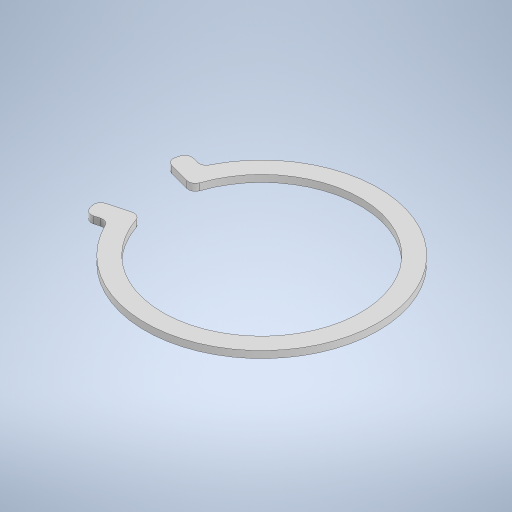
# Autodesk Inventor part: BearingRing
Saved by Autodesk Inventor 2023 (Build 270158030, 158C)
## iProperties
Created: 2024-10-25
Part Number: BearingRing
Material: Generic
Document SubType Name: Modeling
Designer: lvrectanus0
Density: 1 g/cm^3
Appearance: Default
Author: lvrectanus0
Autodesk Inventor part; units mm, degrees
ref_plane "YZ Plane" through (0, 0, 0) normal (1, 0, 0) x (0, 1, 0)
ref_plane "XZ Plane" through (0, 0, 0) normal (0, 1, 0) x (-1, 0, 0)
ref_plane "XY Plane" through (0, 0, 0) normal (0, 0, 1) x (1, 0, 0)
sketch "Sketch1" plane through (0, 0, 0) normal (0, 1, 0) x (-1, 0, 0)
  arc A0 (13.5292, 4.5927) -> (13.5292, -4.5927) centre (0, 0) ccw
  arc A1 (15.0656, 7.4961) -> (15.0656, -7.4961) centre (0, 0) ccw
  line L0 (14.735, -3.9482) -> (16.2541, -4.3553)
  line L1 (0, 0) -> (16.8275, 0) construction
  line L2 (14.735, 3.9482) -> (16.2541, 4.3553)
  line L3 (0, 0) -> (16.8275, 0) construction
  line L4 (16.2541, 4.3553) -> (17.7416, 4.7539)
  line L5 (18.4487, 5.9786) -> (18.309, 6.5002)
  line L6 (17.0842, 7.2073) -> (16.2197, 6.9757)
  line L7 (16.2541, -4.3553) -> (17.7416, -4.7539)
  line L8 (18.4487, -5.9786) -> (18.309, -6.5002)
  line L9 (17.0842, -7.2073) -> (16.2197, -6.9757)
  arc A2 (13.5292, 4.5927) -> (14.735, 3.9482) centre (14.4761, 4.9141) ccw
  arc A3 (17.7416, 4.7539) -> (18.4487, 5.9786) centre (17.4828, 5.7198) ccw
  arc A4 (18.309, 6.5002) -> (17.0842, 7.2073) centre (17.3431, 6.2414) ccw
  arc A5 (15.0656, 7.4961) -> (16.2197, 6.9757) centre (15.9609, 7.9416) ccw
  arc A6 (14.735, -3.9482) -> (13.5292, -4.5927) centre (14.4761, -4.9141) ccw
  arc A7 (18.4487, -5.9786) -> (17.7416, -4.7539) centre (17.4828, -5.7198) ccw
  arc A8 (17.0842, -7.2073) -> (18.309, -6.5002) centre (17.3431, -6.2414) ccw
  arc A9 (16.2197, -6.9757) -> (15.0656, -7.4961) centre (15.9609, -7.9416) ccw
  point P0 (13.8007, 3.6979)
  point P1 (13.8007, -3.6979)
  point P2 (18.7076, 5.0127)
  point P3 (18.0502, 7.4661)
  point P4 (15.4105, 6.7588)
  point P5 (18.7076, -5.0127)
  point P6 (18.0502, -7.4661)
  point P7 (15.4105, -6.7588)
  dimension "d0" = 28.575
  dimension "d1" = 2.54
  dimension "d2" = 15
  dimension "d3" = 15
  dimension "d4" = 2.54
  dimension "d5" = 2.54
  dimension "d6" = 90
  dimension "d7" = 2.54
  dimension "d8" = 2.54
  dimension "d9" = 1
  dimension "d10" = 1
  constraints: 27 point on circle, 20 end point, 16 tangent, 12 point on line, 10 centre point, 6 equal radius, 3 perpendicular, 2 horizontal, 1 coincident
  measures "d0" diameter of A0
  measures "d1" radial gap between concentric circles of A0 A1
  measures "d2" angle of L0 L1
  measures "d3" angle of L3 L2
  measures "d4" distance of L2.end point (18.708, 5.013)
  measures "d5" distance of point (18.708, 5.013) point (18.05, 7.466)
  measures "d6" angle of L6 L5
  measures "d7" distance of L7.start point (18.708, -5.013)
  measures "d8" distance of point (18.708, -5.013) point (18.05, -7.466)
  measures "d9" radius of A2
  measures "d10" radius of A9
extrude "Extrusion1" add sketch "Sketch1" along normal blind 1
body "Solid1"
